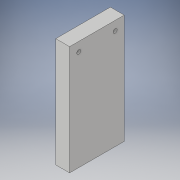
# Autodesk Inventor part: motor stand
Saved by Autodesk Inventor 2019 (Build 230136000, 136)
## iProperties
Created: 2018-11-17
Part Number: motor stand
Material: Generic
Document SubType Name: Modeling
Designer: User
Density: 1 g/cm^3
Appearance: Default
Author: User
Autodesk Inventor part; units mm, degrees
ref_plane "YZ Plane" through (0, 0, 0) normal (1, 0, 0) x (0, 1, 0)
ref_plane "XZ Plane" through (0, 0, 0) normal (0, 1, 0) x (-1, 0, 0)
ref_plane "XY Plane" through (0, 0, 0) normal (0, 0, 1) x (1, 0, 0)
sketch "Sketch1" plane through (0, 0, 0) normal (0, 1, 0) x (-1, 0, 0)
  line L0 (0, 0) -> (9.652, 0)
  line L1 (9.652, 0) -> (9.652, -38.1)
  line L2 (9.652, -38.1) -> (0, -38.1)
  line L3 (0, -38.1) -> (0, 0)
  dimension "d0" = 9.652
  dimension "d1" = 38.1
  constraints: 8 end point, 2 parallel, 1 horizontal, 1 perpendicular
  measures "d0" distance of L1.end L2.end
  measures "d1" distance of L0.end L1.end
extrude "Extrusion1" add sketch "Sketch1" along normal blind 76.2
sketch "Sketch2" plane through (0, 0, 0) normal (1, 0, 0) x (0, 0, -1)
  line L0 (38.1, 0) -> (38.1, 76.2) projected
  line L1 (0, 76.2) -> (38.1, 76.2) projected
  line L2 (0, 0) -> (0, 76.2) projected
  point P0 (6.35, 69.85)
  point P1 (31.75, 69.85)
  dimension "d4" = 6.35
  dimension "d5" = 6.35
  dimension "d6" = 6.35
  dimension "d7" = 6.35
  measures "d4" distance from line of L0 point (31.75, 69.85)
  measures "d5" distance from line of L1 point (31.75, 69.85)
  measures "d6" distance from line of L2 point (6.35, 69.85)
  measures "d7" distance from line of L1 point (6.35, 69.85)
hole "Hole1" at (0, 69.85, -6.35) at (0, 69.85, -31.75) direction (-1, 0, 0) diameter 2.7178 depth 25.4 tip angle 118
equation "\"d5\" = d4"
equation "\"d6\" = d4"
equation "\"d7\" = d4"
body "Solid1"
